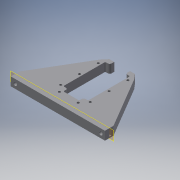
# Autodesk Inventor part: motor_mount
Saved by Autodesk Inventor 2018 (Build 220112000, 112)
## iProperties
Created: 2020-02-21
Part Number: motor_mount
Material: Generic
Document SubType Name: Modeling
Designer: bitbots
Density: 1 g/cm^3
Appearance: Default
Author: bitbots
Autodesk Inventor part; units mm, degrees
ref_plane "YZ Plane" through (0, 0, 0) normal (1, 0, 0) x (0, 1, 0)
ref_plane "XZ Plane" through (0, 0, 0) normal (0, 1, 0) x (-1, 0, 0)
ref_plane "XY Plane" through (0, 0, 0) normal (0, 0, 1) x (1, 0, 0)
sketch "Sketch1" plane through (0, 0, 0) normal (0, 0, 1) x (1, 0, 0)
  line L0 (13.5, -39.75) -> (11.5, -39.75) projected
  arc A0 (11.5, -39.75) -> (9.25, -42) centre (11.5, -42) ccw projected
  line L1 (9.25, -42) -> (9.25, -44) projected
  arc A1 (8.25, -45) -> (9.25, -44) centre (8.25, -44) ccw projected
  line L2 (8.25, -45) -> (-8.25, -45) projected
  arc A2 (-9.25, -44) -> (-8.25, -45) centre (-8.25, -44) ccw projected
  line L3 (-9.25, -44) -> (-9.25, -42) projected
  arc A3 (-9.25, -42) -> (-11.5, -39.75) centre (-11.5, -42) ccw projected
  line L4 (-11.5, -39.75) -> (-13.5, -39.75) projected
  arc A4 (-14.5, -38.75) -> (-13.5, -39.75) centre (-13.5, -38.75) ccw projected
  line L5 (-14.5, -38.75) -> (-14.5, 8.25) projected
  arc A5 (-13.5, 9.25) -> (-14.5, 8.25) centre (-13.5, 8.25) ccw projected
  line L6 (-13.5, 9.25) -> (-11.5, 9.25) projected
  arc A6 (-11.5, 9.25) -> (-9.25, 11.5) centre (-11.5, 11.5) ccw projected
  line L7 (-9.25, 11.5) -> (-9.25, 14.5) projected
  line L8 (-15, 14.5) -> (-9.25, 14.5) projected
  line L9 (-20.1, 8.5) -> (-15, 14.5) projected
  line L10 (-20.1, -44.6) -> (-20.1, 8.5) projected
  line L11 (-15, -50.6) -> (-20.1, -44.6) projected
  line L12 (15, -50.6) -> (-15, -50.6) projected
  line L13 (20.1, -44.6) -> (15, -50.6) projected
  line L14 (20.1, 8.5) -> (20.1, -44.6) projected
  line L15 (15, 14.5) -> (20.1, 8.5) projected
  line L16 (9.25, 14.5) -> (15, 14.5) projected
  line L17 (9.25, 14.5) -> (9.25, 11.5) projected
  arc A7 (9.25, 11.5) -> (11.5, 9.25) centre (11.5, 11.5) ccw projected
  line L18 (11.5, 9.25) -> (13.5, 9.25) projected
  arc A8 (14.5, 8.25) -> (13.5, 9.25) centre (13.5, 8.25) ccw projected
  line L19 (14.5, 8.25) -> (14.5, -38.75) projected
  arc A9 (13.5, -39.75) -> (14.5, -38.75) centre (13.5, -38.75) ccw projected
  circle A10 centre (17.3, 4) radius 1.35 projected
  circle A11 centre (17.3, -18) radius 1.35 projected
  circle A12 centre (11, -47.8) radius 1.35 projected
  circle A13 centre (-17.3, 4) radius 1.35 projected
  circle A14 centre (-17.3, -18) radius 1.35 projected
  circle A15 centre (-11, -47.8) radius 1.35 projected
  circle A16 centre (17.3, -40) radius 1.35 projected
  circle A17 centre (-17.3, -40) radius 1.35 projected
  point P0 (0, 0)
extrude "Extrusion1" add sketch "Sketch1" along normal blind 10
sketch "Sketch2" plane through (-15, -50.6, 0) normal (0, -1, 0) x (1, 0, 0)
  line L0 (0, 0) -> (30, 0) projected
  line L1 (30, 0) -> (30, 10) projected
  line L2 (0, 10) -> (30, 10) projected
  line L3 (0, 0) -> (0, 10) projected
  line L4 (15, 0) -> (70, 0)
  line L5 (70, 0) -> (70, 10)
  line L6 (70, 10) -> (15, 10)
  line L7 (15, 10) -> (15, 0)
  line L8 (15, 0) -> (-40, 0)
  line L9 (-40, 0) -> (-40, 10)
  line L10 (-40, 10) -> (15, 10)
  line L11 (15, 10) -> (15, 0)
  dimension "d2" = 55
  dimension "d3" = 10
  dimension "d4" = 55
  dimension "d5" = 10
  constraints: 16 end point, 4 parallel, 2 horizontal, 2 perpendicular
  measures "d2" distance of L6.end L5.end
  measures "d3" distance of L5.end L4.end
  measures "d4" distance of L9.end L10.end
  measures "d5" distance of L8.end L9.end
extrude "Extrusion2" add sketch "Sketch2" along normal blind 10
sketch "Sketch3" plane through (0, 0, 10) normal (0, 0, 1) x (1, 0, 0)
  circle A0 centre (-17.3, -40) radius 1.35 projected
  circle A1 centre (17.3, -40) radius 1.35 projected
  circle A2 centre (-11, -47.8) radius 1.35 projected
  circle A3 centre (-17.3, -18) radius 1.35 projected
  circle A4 centre (-17.3, 4) radius 1.35 projected
  circle A5 centre (11, -47.8) radius 1.35 projected
  circle A6 centre (17.3, -18) radius 1.35 projected
  circle A7 centre (17.3, 4) radius 1.35 projected
  line L0 (13.5, -39.75) -> (11.5, -39.75) projected
  arc A8 (11.5, -39.75) -> (9.25, -42) centre (11.5, -42) ccw projected
  line L1 (9.25, -42) -> (9.25, -44) projected
  arc A9 (8.25, -45) -> (9.25, -44) centre (8.25, -44) ccw projected
  line L2 (8.25, -45) -> (-8.25, -45) projected
  arc A10 (-9.25, -44) -> (-8.25, -45) centre (-8.25, -44) ccw projected
  line L3 (-9.25, -44) -> (-9.25, -42) projected
  arc A11 (-9.25, -42) -> (-11.5, -39.75) centre (-11.5, -42) ccw projected
  line L4 (-11.5, -39.75) -> (-13.5, -39.75) projected
  arc A12 (-14.5, -38.75) -> (-13.5, -39.75) centre (-13.5, -38.75) ccw projected
  line L5 (-14.5, -38.75) -> (-14.5, 8.25) projected
  arc A13 (-13.5, 9.25) -> (-14.5, 8.25) centre (-13.5, 8.25) ccw projected
  line L6 (-13.5, 9.25) -> (-11.5, 9.25) projected
  arc A14 (-11.5, 9.25) -> (-9.25, 11.5) centre (-11.5, 11.5) ccw projected
  line L7 (-9.25, 11.5) -> (-9.25, 14.5) projected
  line L8 (-9.25, 14.5) -> (-15, 14.5) projected
  line L9 (-15, 14.5) -> (-20.1, 8.5) projected
  line L10 (-20.1, 8.5) -> (-20.1, -44.6) projected
  line L11 (-20.1, -44.6) -> (-15, -50.6) projected
  line L12 (-15, -50.6) -> (-55, -50.6) projected
  line L13 (-55, -50.6) -> (-55, -60.6) projected
  line L14 (55, -60.6) -> (-55, -60.6) projected
  line L15 (55, -50.6) -> (55, -60.6) projected
  line L16 (55, -50.6) -> (15, -50.6) projected
  line L17 (15, -50.6) -> (20.1, -44.6) projected
  line L18 (20.1, -44.6) -> (20.1, 8.5) projected
  line L19 (20.1, 8.5) -> (15, 14.5) projected
  line L20 (15, 14.5) -> (9.25, 14.5) projected
  line L21 (9.25, 14.5) -> (9.25, 11.5) projected
  arc A15 (9.25, 11.5) -> (11.5, 9.25) centre (11.5, 11.5) ccw projected
  line L22 (11.5, 9.25) -> (13.5, 9.25) projected
  arc A16 (14.5, 8.25) -> (13.5, 9.25) centre (13.5, 8.25) ccw projected
  line L23 (14.5, 8.25) -> (14.5, -38.75) projected
  arc A17 (13.5, -39.75) -> (14.5, -38.75) centre (13.5, -38.75) ccw projected
  line L24 (-20.1, 8.5) -> (-55, -50.6)
  line L25 (20.1, -44.6) -> (20.1, 8.5) projected
  line L26 (15, -50.6) -> (55, -50.6) projected
  line L27 (20.1, 8.5) -> (55, -50.6)
  point P0 (0, 0)
  constraints: 4 end point
extrude "Extrusion3" add sketch "Sketch3" against normal blind 10 contours L27 L16 L17 L18 | L24 L10 L11 L12
sketch "Sketch4" plane through (-15, -60.6, 0) normal (0, -1, 0) x (1, 0, 0)
  line L0 (15, 0) -> (15, 5)
  line L1 (15, 0) -> (20, 0) construction
  line L2 (15, 5) -> (-35, 5)
  line L3 (15, 5) -> (65, 5)
  line L4 (15, 5) -> (65, 5) construction
  circle A0 centre (-35, 5) radius 2.1
  circle A1 centre (65, 5) radius 2.1
  dimension "d10" = 5
  dimension "d11" = 90
  dimension "d12" = 50
  dimension "d13" = 90
  dimension "d14" = 50
  dimension "d15" = 0
  dimension "d16" = 4.2
  dimension "d17" = 4.2
  constraints: 10 end point, 3 horizontal, 2 centre point, 2 coincident, 2 equal length, 1 perpendicular, 1 vertical
  measures "d10" distance of L0.start L0.end
  measures "d11" angle of L1 L0
  measures "d12" distance of L0.end L2.end
  measures "d13" angle of L2 L0
  measures "d14" distance of L0.end L3.end
  measures "d15" distance between parallel lines of L3 L4
  measures "d16" diameter of A0
  measures "d17" diameter of A1
extrude "Extrusion4" cut sketch "Sketch4" against normal blind 10
ref_plane "Work Plane1" through (-15, -55.6, 0) normal (0, -1, 0) x (1, 0, 0)
sketch "Sketch5" plane through (-15, -55.6, 0) normal (0, -1, 0) x (1, 0, 0)
  circle A0 centre (-35, 5) radius 2.1 projected
  circle A1 centre (65, 5) radius 2.1 projected
  line L0 (-38.6, 8.6) -> (-31.4, 8.6)
  line L1 (-31.4, 8.6) -> (-31.4, 1.4)
  line L2 (-31.4, 1.4) -> (-38.6, 1.4)
  line L3 (-38.6, 1.4) -> (-38.6, 8.6)
  line L4 (-38.6, 8.6) -> (-31.4, 1.4)
  line L5 (-31.4, 8.6) -> (-38.6, 1.4)
  line L6 (61.4, 8.6) -> (68.6, 8.6)
  line L7 (68.6, 8.6) -> (68.6, 1.4)
  line L8 (68.6, 1.4) -> (61.4, 1.4)
  line L9 (61.4, 1.4) -> (61.4, 8.6)
  line L10 (61.4, 8.6) -> (68.6, 1.4)
  line L11 (68.6, 8.6) -> (61.4, 1.4)
  line L12 (70, 0) -> (70, 10) projected
  line L13 (68.6, 1.4) -> (70, 1.4)
  line L14 (70, 1.4) -> (70, 8.6)
  line L15 (70, 8.6) -> (68.6, 8.6)
  line L16 (68.6, 8.6) -> (68.6, 1.4)
  line L17 (-40, 10) -> (-40, 0) construction
  line L18 (-38.6, 8.6) -> (-40, 8.6)
  line L19 (-40, 8.6) -> (-40, 1.4)
  line L20 (-40, 1.4) -> (-38.6, 1.4)
  line L21 (-38.6, 1.4) -> (-38.6, 8.6)
  point P0 (15, 0)
  dimension "d21" = 7.2
  dimension "d22" = 7.2
  dimension "d23" = 7.2
  dimension "d24" = 7.2
  constraints: 40 end point, 8 parallel, 4 horizontal, 4 midpoint, 4 perpendicular, 2 point on line
  measures "d21" distance of L1.end L2.end
  measures "d22" distance of L0.end L1.end
  measures "d23" distance of L7.end L8.end
  measures "d24" distance of L6.end L7.end
extrude "Extrusion5" cut sketch "Sketch5" against normal blind 2.5
body "Solid1"
